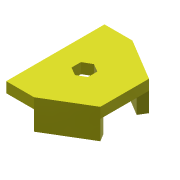
# Autodesk Inventor part: 30_Cube_Z_Focus_Drylin_NEMA_slide_part1
Saved by Autodesk Inventor 2019.4 (Build 234330000, 330)
## iProperties
Created: 2021-05-05
Part Number: 30_Cube_Z_Focus_Drylin_NEMA_slide_part1
Material: Generic
Document SubType Name: Modeling
Designer: diederichbenedict
Density: 1 g/cm^3
Appearance: Smooth - Yellow
Author: diederichbenedict
Autodesk Inventor part; units mm, degrees
ref_plane "YZ Plane" through (0, 0, 0) normal (1, 0, 0) x (0, 1, 0)
ref_plane "XZ Plane" through (0, 0, 0) normal (0, 1, 0) x (-1, 0, 0)
ref_plane "XY Plane" through (0, 0, 0) normal (0, 0, 1) x (1, 0, 0)
sketch "Sketch1" plane through (0, 0, 0) normal (0, 1, 0) x (-1, 0, 0)
  line L0 (-13.5, -12.4952) -> (9.75, -12.4952)
  line L1 (9.75, -12.4952) -> (9.75, 12.4952)
  line L2 (9.75, 12.4952) -> (-13.5, 12.4952)
  line L3 (-13.5, 12.4952) -> (-13.5, -12.4952)
  circle A0 centre (-7.5, 0) radius 4
  circle A1 centre (3.75, -6.4952) radius 4
  circle A2 centre (3.75, 6.4952) radius 4
  line L4 (-2.75, -1.5877) -> (-2.75, 1.5877)
  line L5 (-2.75, 1.5877) -> (0, 3.1754)
  line L6 (0, 3.1754) -> (2.75, 1.5877)
  line L7 (2.75, 1.5877) -> (2.75, -1.5877)
  line L8 (2.75, -1.5877) -> (0, -3.1754)
  line L9 (0, -3.1754) -> (-2.75, -1.5877)
  circle A3 centre (0, 0) radius 7.5 construction
  dimension "d11" = 15
  dimension "d2" = 8
  dimension "d6" = 360
  dimension "d8" = 6
  dimension "d9" = 6
  dimension "d10" = 5.5
  dimension "d12" = 6
  dimension "d13" = 6
  constraints: 20 end point, 3 centre point, 3 parallel, 2 coincident, 1 horizontal, 1 horizontal alignment, 1 perpendicular, 22 other
  measures "d2" diameter of A0
  measures "d8" distance from line of A2.centre L1
  measures "d9" distance from line of L3 A0.centre
  measures "d10" distance between parallel lines of L4 L7
  measures "d12" distance from line of L2 A2.centre
  measures "d13" distance from line of L0 A1.centre
extrude "Extrusion1" add sketch "Sketch1" along normal blind 3
sketch "Sketch2" plane through (0, 3, 0) normal (0, 1, 0) x (1, 0, 0)
  circle A0 centre (-3.75, -6.4952) radius 4 projected
  circle A1 centre (-3.75, 6.4952) radius 4 projected
  circle A2 centre (7.5, 0) radius 4 projected
  line L0 (2.75, -1.5877) -> (0, -3.1754) projected
  line L1 (0, -3.1754) -> (-2.75, -1.5877) projected
  line L2 (-2.75, -1.5877) -> (-2.75, 1.5877) projected
  line L3 (-2.75, 1.5877) -> (0, 3.1754) projected
  line L4 (0, 3.1754) -> (2.75, 1.5877) projected
  line L5 (2.75, 1.5877) -> (2.75, -1.5877) projected
  line L6 (13.5, 12.4952) -> (-9.75, 12.4952) projected
  line L7 (-9.75, 12.4952) -> (-9.75, -12.4952) projected
  line L8 (-9.75, -12.4952) -> (13.5, -12.4952) projected
  line L9 (13.5, -12.4952) -> (13.5, 12.4952) projected
  circle A3 centre (0, 0) radius 1.75
  dimension "d16" = 3.5
  constraints: 1 centre point, 1 coincident
  measures "d16" diameter of A3
extrude "Extrusion2" add sketch "Sketch2" along normal blind 0.5 contours A0 | A1 | A2 | L9 L8 L7 L6
sketch "Sketch3" plane through (0, 0, 0) normal (0, -1, 0) x (1, 0, 0)
  circle A0 centre (-3.75, 6.4952) radius 4 projected
  circle A1 centre (-3.75, -6.4952) radius 4 projected
  circle A2 centre (7.5, 0) radius 4 projected
  line L0 (0, 3.1754) -> (2.75, 1.5877) projected
  line L1 (2.75, 1.5877) -> (2.75, -1.5877) projected
  line L2 (2.75, -1.5877) -> (0, -3.1754) projected
  line L3 (0, -3.1754) -> (-2.75, -1.5877) projected
  line L4 (-2.75, -1.5877) -> (-2.75, 1.5877) projected
  line L5 (-2.75, 1.5877) -> (0, 3.1754) projected
  line L6 (13.5, -12.4952) -> (-9.75, -12.4952) projected
  line L7 (13.5, 12.4952) -> (13.5, -12.4952) projected
  line L8 (-9.75, 12.4952) -> (13.5, 12.4952) projected
  line L9 (-9.75, -12.4952) -> (-9.75, 12.4952) construction
  line L10 (-1.5, 12.4952) -> (13.5, 3.4952)
  line L11 (13.5, 12.4952) -> (13.5, -12.4952) projected
  line L12 (13.5, -3.4952) -> (-1.5, -12.4952)
  point P0 (0, 0)
  dimension "d19" = 9
  dimension "d20" = 9
  dimension "d21" = 15
  dimension "d22" = 15
  constraints: 4 end point, 4 point on line
  measures "d19" distance from line of L8 L10.end
  measures "d20" distance from line of L6 L12.start
  measures "d21" distance from line of L12.end L7
  measures "d22" distance from line of L7 L10.start
extrude "Extrusion3" cut sketch "Sketch3" against normal through all contours L6 L12 L7 | L7 L10 L8
sketch "Sketch4" plane through (0, 0, 0) normal (0, -1, 0) x (1, 0, 0)
  line L0 (0, 3.1754) -> (2.75, 1.5877) projected
  line L1 (-2.75, 1.5877) -> (0, 3.1754) projected
  line L2 (-2.75, -1.5877) -> (-2.75, 1.5877) projected
  line L3 (0, -3.1754) -> (-2.75, -1.5877) construction
  line L4 (2.75, -1.5877) -> (0, -3.1754) projected
  line L5 (3.5876, -2.6244) -> (-4.4124, -2.6244) projected
  circle A0 centre (0, 0) radius 1.6 projected
  line L6 (2.75, 1.5877) -> (2.75, -1.5877) projected
  line L7 (-2.65, -1.53) -> (-2.65, 1.53)
  line L8 (-2.65, 1.53) -> (0, 3.06)
  line L9 (0, 3.06) -> (2.65, 1.53)
  line L10 (2.65, 1.53) -> (2.65, -1.53)
  line L11 (2.65, -1.53) -> (0, -3.06)
  line L12 (0, -3.06) -> (-2.65, -1.53)
  point P0 (0, 0)
  dimension "d34" = 0.1
  constraints: 12 end point, 5 other
  measures "d34" distance between parallel lines of L3 L12
extrude "Extrusion4" [suppressed]
sketch "Sketch5" plane through (0, 0, 0) normal (0, -1, 0) x (1, 0, 0)
  line L0 (13.5, 3.4952) -> (-1.5, 12.4952) projected
  line L1 (-9.75, 12.4952) -> (-1.5, 12.4952) projected
  line L2 (-9.75, -12.4952) -> (-9.75, 12.4952) projected
  line L3 (-1.5, -12.4952) -> (-9.75, -12.4952) projected
  line L4 (-1.5, -12.4952) -> (13.5, -3.4952) projected
  line L5 (13.5, 3.4952) -> (13.5, -3.4952) projected
  circle A0 centre (-3.75, 6.4952) radius 4 projected
  circle A1 centre (-3.75, -6.4952) radius 4 projected
  circle A2 centre (7.5, 0) radius 4 projected
  line L6 (17.5, -5.76) -> (-0.3921, -16.4952)
  line L7 (-0.3921, -16.4952) -> (-13.75, -16.4952)
  line L8 (-13.75, -16.4952) -> (-13.75, 16.4952)
  line L9 (-13.75, 16.4952) -> (-0.3921, 16.4952)
  line L10 (-0.3921, 16.4952) -> (17.5, 5.76)
  line L11 (17.5, 5.76) -> (17.5, -5.76)
  line L12 (13.5, -3.4952) -> (13.5, -8.16)
  line L13 (13.5, 3.4118) -> (13.5, 8.16)
  line L14 (-1.5, -12.4952) -> (-9.75, -12.4952) projected
  line L15 (-9.75, -12.4952) -> (-9.75, -16.4952)
  line L16 (-9.75, 12.4952) -> (-1.5, 12.4952) projected
  line L17 (-9.75, 12.4952) -> (-9.75, 16.4952)
  line L18 (-1.5, -12.4952) -> (13.5, -3.4952) projected
  line L19 (13.5, -3.4952) -> (-1.5, -12.4952)
  line L20 (-1.5, -12.4952) -> (-9.75, -12.4952)
  line L21 (-9.75, -12.4952) -> (-9.75, 12.4952) projected
  line L22 (-9.75, 12.4952) -> (-1.5, 12.4952)
  line L23 (13.5, 3.4952) -> (-1.5, 12.4952) projected
  line L24 (13.5, 3.4952) -> (-1.5, 12.4952)
  line L25 (13.5, -3.4952) -> (13.5, 3.4118)
  point P0 (0, 0)
  dimension "d27" = 4
  constraints: 30 end point, 6 point on line, 4 collinear, 2 perpendicular, 2 vertical, 5 other
  measures "d27" distance between parallel lines of L4 L6
extrude "Extrusion5" add sketch "Sketch5" against normal up to surface (3.5 mm away) contours L0 L1 L17 L9 L10 L13 | L12 L6 L7 L15 L3 L4
sketch "Sketch6" plane through (0, 3.5, 0) normal (0, 1, 0) x (1, 0, 0)
  line L0 (0, -3.1754) -> (-2.75, -1.5877) projected
  line L1 (-2.75, -1.5877) -> (-2.75, 1.5877) projected
  line L2 (-2.75, 1.5877) -> (0, 3.1754) projected
  line L3 (0, 3.1754) -> (2.75, 1.5877) projected
  line L4 (2.75, 1.5877) -> (2.75, -1.5877) projected
  line L5 (2.75, -1.5877) -> (0, -3.1754) projected
  line L6 (13.5, -8.16) -> (13.5, 8.16) projected
  line L7 (-0.3921, 16.4952) -> (13.5, 8.16) projected
  line L8 (-9.75, 16.4952) -> (-0.3921, 16.4952) projected
  line L9 (-9.75, -16.4952) -> (-9.75, 16.4952) projected
  line L10 (-0.3921, -16.4952) -> (-9.75, -16.4952) projected
  line L11 (13.5, -8.16) -> (-0.3921, -16.4952) projected
  line L12 (13.5, 8.16) -> (-0.3921, 16.4952)
  line L13 (-0.3921, 16.4952) -> (-1.9356, 13.9227)
  line L14 (-1.9356, 13.9227) -> (11.9565, 5.5875)
  line L15 (11.9565, 5.5875) -> (13.5, 8.16)
  line L16 (13.5, -8.16) -> (13.5, 8.16) projected
  line L17 (13.5, -8.16) -> (-0.3921, -16.4952)
  line L18 (-0.3921, -16.4952) -> (-1.9356, -13.9227)
  line L19 (-1.9356, -13.9227) -> (11.9565, -5.5875)
  line L20 (11.9565, -5.5875) -> (13.5, -8.16)
  point P0 (0, 0)
  dimension "d30" = 3
  dimension "d31" = 3
  constraints: 16 end point, 5 equal length, 2 perpendicular
  measures "d30" distance of L13.end L7.start
  measures "d31" distance of L10.start L18.end
extrude "Extrusion6" add sketch "Sketch6" against normal blind 10 contours L11 L18 L19 L20 | L15 L14 L13 L7
body "Solid1"
